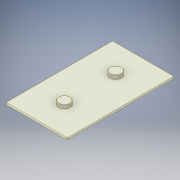
# Autodesk Inventor part: Bottom Surface
Saved by Autodesk Inventor 2019.4 (Build 234330000, 330)
## iProperties
Created: 2021-03-04
Part Number: Bottom Surface
Material: Polytetrafluoroethylene
Document SubType Name: Modeling
Designer: caleb
Density: 2.02 g/cm^3
Appearance: Smooth - Ivory
Author: caleb
Autodesk Inventor part; units mm, degrees
ref_plane "YZ Plane" through (0, 0, 0) normal (1, 0, 0) x (0, 1, 0)
ref_plane "XZ Plane" through (0, 0, 0) normal (0, 1, 0) x (-1, 0, 0)
ref_plane "XY Plane" through (0, 0, 0) normal (0, 0, 1) x (1, 0, 0)
sketch "Sketch1" plane through (0, 0, 0) normal (0, 1, 0) x (-1, 0, 0)
  line L0 (-13.15, 22.85) -> (13.15, 22.85)
  line L1 (13.15, 22.85) -> (13.15, -22.85)
  line L2 (13.15, -22.85) -> (-13.15, -22.85)
  line L3 (-13.15, -22.85) -> (-13.15, 22.85)
  line L4 (-13.15, 22.85) -> (13.15, -22.85) construction
  line L5 (13.15, 22.85) -> (-13.15, -22.85) construction
  point P0 (0, 0)
  dimension "d0" = 45.7
  dimension "d1" = 26.3
  constraints: 12 end point, 2 midpoint, 2 parallel, 1 horizontal, 1 perpendicular
  measures "d0" distance of L0.end L1.end
  measures "d1" distance of L0.start L0.end
extrude "Extrusion1" add sketch "Sketch1" along normal blind 2
sketch "Sketch2" plane through (0, 2, 0) normal (0, 1, 0) x (1, 0, 0)
  circle A0 centre (0, -11) radius 2.5
  circle A1 centre (0, 11) radius 2.5
  point P0 (0, 0)
  dimension "d4" = 5
  dimension "d5" = 5
  dimension "d6" = 11
  dimension "d7" = 11
  constraints: 2 centre point
  measures "d4" diameter of A0
  measures "d5" diameter of A1
  measures "d6" distance of point (0, 0) A0.centre
  measures "d7" distance of point (0, 0) A1.centre
extrude "Extrusion2" add sketch "Sketch2" along normal blind 1.5
fillet "Fillet1" radius 0.2 1 edges at (-2.5, 3.5, 11)
fillet "Fillet2" radius 0.2 1 edges at (-2.5, 3.5, -11)
sketch "Sketch3" plane through (0, 0, 0) normal (0, -1, 0) x (1, 0, 0)
  line L0 (13.15, -22.85) -> (-13.15, -22.85) projected
  line L1 (-13.15, 22.85) -> (13.15, 22.85)
  line L2 (13.15, 22.85) -> (13.15, -22.85)
  line L3 (13.15, -22.85) -> (-13.15, -22.85)
  line L4 (-13.15, -22.85) -> (-13.15, 22.85)
  line L5 (-13.15, 22.85) -> (13.15, -22.85) construction
  line L6 (13.15, 22.85) -> (-13.15, -22.85) construction
  line L7 (-9.9, 20.3) -> (9.9, 20.3)
  line L8 (9.9, 20.3) -> (9.9, -20.3)
  line L9 (9.9, -20.3) -> (-9.9, -20.3)
  line L10 (-9.9, -20.3) -> (-9.9, 20.3)
  line L11 (-9.9, 20.3) -> (9.9, -20.3) construction
  line L12 (9.9, 20.3) -> (-9.9, -20.3) construction
  point P0 (0, 0)
  dimension "d12" = 19.8
  dimension "d13" = 40.6
  constraints: 24 end point, 4 midpoint, 4 parallel, 2 horizontal, 2 perpendicular
  measures "d12" distance of L7.start L7.end
  measures "d13" distance of L7.end L8.end
extrude "Extrusion3" cut sketch "Sketch3" against normal blind 1
fillet "Fillet3" radius 0.2 16 edges at (13.15, 1, 0) (9.9, 0, 0) (9.9, 0.5, 20.3) (0, 0, 20.3) (0, 1, 22.85) (-9.9, 0, 0) (-13.15, 1, 0) (-9.9, 0.5, -20.3) (0, 0, -20.3) (9.9, 0.5, -20.3) (0, 1, -22.85) (-9.9, 0.5, 20.3) (-13.15, 1.5, 22.85) (-13.15, 1.5, -22.85) (13.15, 1.5, -22.85) (13.15, 1.5, 22.85)
body "Solid1"
